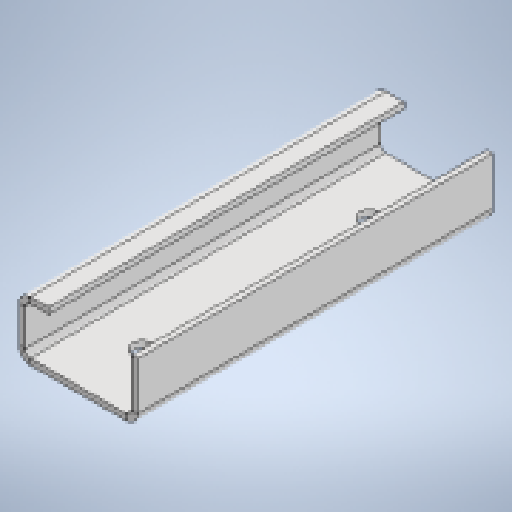
# Autodesk Inventor part: PNS 2114 cyclone plate
Saved by Autodesk Inventor 2025.3 (Build 293356030, 356C)
## iProperties
Created: 2025-09-12
Part Number: PNS 2114 cyclone plate
Material: Stainless Steel
Document SubType Name: Sheet Metal
Designer: admin
Mass: 341.83 g
Surface Area: 302.343 cm^2
Volume: 42.7288 cm^3
Density: 8 g/cm^3
Sheet Metal Rule: AISI304 2mm Die16
Sheet Metal Width: 80,000 mm
Sheet Metal Length: 180,000 mm
Sheet Metal Area: 14400,000 mm^2
Appearance: Default
Flat Pattern Width: 8 cm
Flat Pattern Length: 18 cm
Flat Pattern Area: 144 cm^2
Author: admin
Autodesk Inventor part; units mm, degrees
ref_plane "YZ Plane" through (0, 0, 0) normal (1, 0, 0) x (0, 1, 0)
ref_plane "XZ Plane" through (0, 0, 0) normal (0, 1, 0) x (-1, 0, 0)
ref_plane "XY Plane" through (0, 0, 0) normal (0, 0, 1) x (1, 0, 0)
sketch "Sketch1" plane through (0, 0, 0) normal (0, 0, 1) x (1, 0, 0)
  line L0 (-40, -90) -> (40, -90)
  line L1 (40, -90) -> (40, 90)
  line L2 (40, 90) -> (-40, 90)
  line L3 (-40, 90) -> (-40, -90)
  line L4 (-40, -90) -> (40, 90) construction
  line L5 (40, -90) -> (-40, 90) construction
  point P0 (0, 0)
  dimension "d154" = 80
  dimension "d155" = 180
  measures "d154" distance of L1.end L2.end
  measures "d155" distance of L0.end L1.end
extrude "Plate5" add sketch "Sketch1" along normal blind 3
sketch "Sketch7" plane through (0, 0, 3) normal (0, 0, 1) x (1, 0, 0)
  circle A0 centre (0, -57.5) radius 5
  circle A1 centre (0, 57.5) radius 5
  line L0 (0, 0) -> (-40, 0) construction
  line L1 (-40, 90) -> (-40, -90) construction
  dimension "d157" = 115
  dimension "d158" = 10
  constraints: 2 centre point, 2 end point, 1 midpoint, 1 vertical alignment, 1 other
  measures "d157" distance of A1.centre A0.centre
  measures "d158" diameter of A0
extrude "Cut1" cut sketch "Sketch7" against normal blind 3
body "Solid3"
